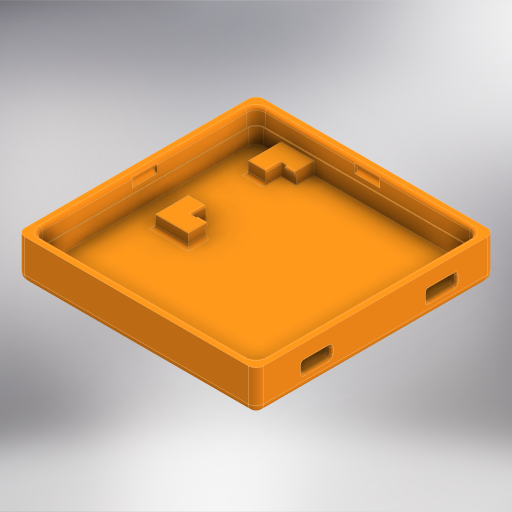
# Autodesk Inventor part: Bottom Plate
Saved by Autodesk Inventor 2024 (Build 280153000, 153)
## iProperties
Created: 2026-05-15
Part Number: Bottom Plate
Material: Generic
Document SubType Name: Modeling
Designer: Satyajit
Density: 1 g/cm^3
Appearance: Orange
Author: Satyajit
Autodesk Inventor part; units mm, degrees
ref_plane "YZ Plane" through (0, 0, 0) normal (1, 0, 0) x (0, 1, 0)
ref_plane "XZ Plane" through (0, 0, 0) normal (0, 1, 0) x (-1, 0, 0)
ref_plane "XY Plane" through (0, 0, 0) normal (0, 0, 1) x (1, 0, 0)
sketch "Sketch1" plane through (0, 0, 0) normal (0, 1, 0) x (-1, 0, 0)
  line L0 (35, -35) -> (-35, -35)
  line L1 (-35, -35) -> (-35, 35)
  line L2 (-35, 35) -> (35, 35)
  line L3 (35, 35) -> (35, -35)
  line L4 (35, -35) -> (-35, 35) construction
  line L5 (-35, -35) -> (35, 35) construction
  line L6 (-38, 38) -> (-38, -38)
  line L7 (-38, -38) -> (38, -38)
  line L8 (38, -38) -> (38, 38)
  line L9 (38, 38) -> (-38, 38)
  point P0 (0, 0)
  dimension "d0" = 70
  dimension "d1" = 3
  constraints: 20 end point, 4 parallel, 3 perpendicular, 2 midpoint, 1 horizontal, 3 other
  measures "d0" distance of L1.end L2.end
  measures "d1" distance between parallel lines of L1 L6
extrude "Extrusion1" add sketch "Sketch1" against normal blind 3 contours L0 L1 L2 L3 | L9 L8 L7 L6
extrude "Extrusion2" add sketch "Sketch1" along normal blind 10
sketch "Sketch2" plane through (0, 0, 0) normal (0, 1, 0) x (1, 0, 0)
  line L0 (-21, 29) -> (36, 29)
  line L1 (36, 29) -> (36, 1)
  line L2 (36, 1) -> (-21, 1)
  line L3 (-21, 1) -> (-21, 29) construction
  line L4 (-21, 29) -> (36, 1) construction
  line L5 (36, 29) -> (-21, 1) construction
  line L6 (-21, 24.15) -> (-27, 24.15) construction
  line L7 (-27, 24.15) -> (-27, 5.85) construction
  line L8 (-27, 5.85) -> (-21, 5.85) construction
  line L9 (35, 35) -> (35, -35) projected
  line L10 (-35, -35) -> (-35, 35) construction
  line L11 (38, 38) -> (38, -38) projected
  line L12 (-35, 35) -> (35, 35) projected
  line L13 (-21.4, 24.55) -> (-21.4, 29.4)
  line L14 (-21.4, 29.4) -> (-16.55, 29.4)
  line L15 (-16.55, 29.4) -> (-16.55, 35)
  line L16 (-21.4, 24.55) -> (-27, 24.55)
  line L17 (-27, 24.55) -> (-27, 35)
  line L18 (7.5, 15) -> (-27, 15) construction
  line L19 (-21.4, 5.45) -> (-21.4, 0.6)
  line L20 (-21.4, 0.6) -> (-16.55, 0.6)
  line L21 (-16.55, 0.6) -> (-16.55, -5)
  line L22 (-21.4, 5.45) -> (-27, 5.45)
  line L23 (-27, 5.45) -> (-27, -5)
  line L24 (-27, -5) -> (-16.55, -5)
  line L25 (35, 0.5) -> (36, 0.5)
  line L26 (36, 0.5) -> (36, 1)
  line L27 (35, 29) -> (35, 29.5)
  line L28 (35, 29.5) -> (36, 29.5)
  line L29 (36, 29.5) -> (36, 29)
  point P0 (0, 0)
  point P1 (40, 34)
  point P2 (35, 1)
  dimension "d16" = 57
  dimension "d17" = 28
  dimension "d18" = 6
  dimension "d19" = 18.3
  dimension "d26" = 2
  dimension "d27" = 6
  dimension "d28" = 0.4
  dimension "d29" = 0.4
  dimension "d30" = 0.4
  dimension "d35" = 0.5
  constraints: 52 end point, 11 perpendicular, 8 point on line, 6 symmetric about line, 4 horizontal, 3 midpoint, 2 collinear, 2 parallel, 1 horizontal alignment, 1 vertical, 1 other
  measures "d16" distance of L0.start L0.end
  measures "d17" distance of L0.end L1.end
  measures "d18" distance between parallel lines of L3 L7
  measures "d19" distance of L6.end L7.end
  measures "d26" distance between parallel lines of L11 L1
  measures "d27" distance between parallel lines of L12 L0
  measures "d28" distance between parallel lines of L6 L16
  measures "d29" distance between parallel lines of L13 L3
  measures "d30" distance between parallel lines of L14 L0
  measures "d35" distance of L28.end L0.end
extrude "Extrusion3" add sketch "Sketch2" along normal blind 4 contours L12 L15 L14 L13 L16 L17 | L19 L20 L21 L24 L23 L22
extrude "Extrusion4" cut sketch "Sketch2" along normal blind 6 contours L9 L28 L29 L0 | L0 L1 L2 L9 | L2 L26 L25 L9
sketch "Sketch3" plane through (36, 0, -29.5) normal (-1, 0, 0) x (0, 0, 1)
  line L0 (29, 0) -> (0, 0) projected
  line L1 (29, 0) -> (29, 6) projected
  line L2 (29, 6) -> (0, 6) projected
  line L3 (0, 0) -> (0, 6) projected
  line L4 (4.35, 1.45) -> (12.65, 1.45)
  line L5 (13.15, 1.95) -> (13.15, 4.45)
  line L6 (12.65, 4.95) -> (4.35, 4.95)
  line L7 (3.85, 4.45) -> (3.85, 1.95)
  line L8 (3.85, 1.45) -> (13.15, 4.95) construction
  line L9 (13.15, 1.45) -> (3.85, 4.95) construction
  line L10 (14.5, 0) -> (14.5, 6) construction
  line L11 (24.65, 1.45) -> (16.35, 1.45)
  line L12 (15.85, 1.95) -> (15.85, 4.45)
  line L13 (16.35, 4.95) -> (24.65, 4.95)
  line L14 (25.15, 4.45) -> (25.15, 1.95)
  line L15 (25.15, 1.45) -> (15.85, 4.95) construction
  line L16 (15.85, 1.45) -> (25.15, 4.95) construction
  arc A0 (3.85, 1.95) -> (4.35, 1.45) centre (4.35, 1.95) ccw
  arc A1 (4.35, 4.95) -> (3.85, 4.45) centre (4.35, 4.45) ccw
  arc A2 (13.15, 4.45) -> (12.65, 4.95) centre (12.65, 4.45) ccw
  arc A3 (12.65, 1.45) -> (13.15, 1.95) centre (12.65, 1.95) ccw
  arc A4 (15.85, 1.95) -> (16.35, 1.45) centre (16.35, 1.95) ccw
  arc A5 (16.35, 4.95) -> (15.85, 4.45) centre (16.35, 4.45) ccw
  arc A6 (25.15, 4.45) -> (24.65, 4.95) centre (24.65, 4.45) ccw
  arc A7 (24.65, 1.45) -> (25.15, 1.95) centre (24.65, 1.95) ccw
  line L17 (44.4, 1.45) -> (52.1, 1.45)
  line L18 (52.9, 2.25) -> (52.9, 4.15)
  line L19 (52.1, 4.95) -> (44.4, 4.95)
  line L20 (43.6, 4.15) -> (43.6, 2.25)
  line L21 (43.6, 1.45) -> (52.9, 4.95) construction
  line L22 (52.9, 1.45) -> (43.6, 4.95) construction
  arc A8 (43.6, 2.25) -> (44.4, 1.45) centre (44.4, 2.25) ccw
  arc A9 (44.4, 4.95) -> (43.6, 4.15) centre (44.4, 4.15) ccw
  arc A10 (52.9, 4.15) -> (52.1, 4.95) centre (52.1, 4.15) ccw
  arc A11 (52.1, 1.45) -> (52.9, 2.25) centre (52.1, 2.25) ccw
  line L23 (29, 0) -> (67.5, 0)
  line L24 (67.5, -3) -> (67.5, 10) projected
  line L25 (42.25, 0) -> (42.25, 6)
  line L26 (42.25, 6) -> (54.25, 6)
  line L27 (54.25, 6) -> (54.25, 0)
  point P0 (29.5, 0)
  point P1 (8.5, 3.2)
  point P2 (20.5, 3.2)
  point P3 (20.5, 3.2)
  point P4 (48.25, 3.2)
  point P5 (48.25, 0)
  point P6 (48.25, 6)
  dimension "d36" = 9.3
  dimension "d37" = 3.5
  dimension "d40" = 12
  dimension "d41" = 3.2
  dimension "d42" = 0.5
  dimension "d45" = 9.3
  dimension "d46" = 3.5
  dimension "d47" = 0.8
  dimension "d48" = 12
  constraints: 46 end point, 27 point on line, 24 point on circle, 24 tangent, 12 centre point, 10 equal radius, 9 midpoint, 5 parallel, 5 symmetric about line, 4 perpendicular, 3 horizontal, 2 vertical alignment, 1 horizontal alignment, 1 vertical
  measures "d36" distance of L8.end L9.end
  measures "d37" distance of L9.start L8.end
  measures "d40" distance of point (8.5, 3.2) point (20.5, 3.2)
  measures "d41" distance from line of L0 point (8.5, 3.2)
  measures "d42" radius of A0
  measures "d45" distance of L21.end L22.end
  measures "d46" distance of L22.start L21.end
  measures "d47" radius of A8
  measures "d48" distance between parallel lines of L27 L25
extrude "Extrusion5" cut sketch "Sketch3" against normal blind 6 contours A0 L7 A1 L6 A2 L5 A3 L4 | A8 L20 A9 L19 A10 L18 A11 L17
extrude "Extrusion6" cut sketch "Sketch3" along normal blind 6 contours A8 L20 A9 L19 A10 L18 A11 L17 | L25 L26 L27 L23
sketch "Sketch4" plane through (0, 4, 0) normal (0, 1, 0) x (1, 0, 0)
  line L0 (-16.55, 0.6) -> (-21.4, 0.6) projected
  line L1 (-21.4, 0.6) -> (-21.4, 5.45) projected
  line L2 (-16.55, -5) -> (-16.55, 0.6) projected
  line L3 (-16.55, 0.6) -> (-16.55, 1.3)
  line L4 (-16.55, 1.3) -> (-19.55, 1.3)
  line L5 (-19.55, 1.3) -> (-19.55, 0.6)
  line L6 (-21.4, 5.45) -> (-27, 5.45) projected
  line L7 (-27, 35) -> (-27, 24.55) projected
  line L8 (-27, 5.45) -> (-27, 24.55) construction
  line L9 (-27, 15) -> (0, 15) construction
  line L10 (-27, 24.55) -> (-21.4, 24.55) projected
  line L11 (-21.4, 24.55) -> (-21.4, 29.4) projected
  line L12 (-21.4, 29.4) -> (-16.55, 29.4) projected
  line L13 (-16.55, 29.4) -> (-16.55, 28.7)
  line L14 (-16.55, 28.7) -> (-19.55, 28.7)
  line L15 (-19.55, 28.7) -> (-19.55, 29.4)
  point P0 (0, 0)
  point P1 (-19.55, 29.4)
  dimension "d51" = 0.7
  dimension "d52" = 3
  constraints: 16 end point, 3 symmetric about line, 2 perpendicular, 2 vertical, 1 horizontal, 1 midpoint, 1 point on line, 1 vertical alignment
  measures "d51" distance of L0.start L3.end
  measures "d52" distance of L3.end L4.end
extrude "Extrusion7" add sketch "Sketch4" against normal blind 1
fillet "Fillet1" radius 0.5 4 edges at (-18.05, 4, -1.3) (-18.05, 3, -1.3) (-18.05, 4, -28.7) (-18.05, 3, -28.7)
fillet "Fillet2" radius 1 2 edges at (-18.05, 3, -0.6) (-18.05, 3, -29.4)
fillet "Fillet3" radius 0.5 8 edges at (-21.4, 4, -26.975) (-21.4, 4, -3.025) (35, 3, -29.5) (35, 6, -15) (35, 3, -0.5) (35, 3, 12.75) (35, 6, 18.75) (35, 3, 24.75)
fillet "Fillet4" radius 2.5 8 edges at (35, 5, -35) (38, 3.5, -38) (38, 3.5, 38) (35, 5, 35) (-38, 3.5, -38) (-38, 3.5, 38) (-35, 5, 35) (-35, 5, -35)
fillet "Fillet6" radius 1 5 edges at (-21.775, 0, 5) (-27, 0, -0.225) (-24.2, 0, -24.55) (-27, 0, -29.775) (-16.55, 0, 2.2)
fillet "Fillet7" radius 2.5 8 edges at (37.2678, -3, 37.2678) (0, -3, 38) (-37.2678, -3, 37.2678) (-38, -3, 0) (-37.2678, -3, -37.2678) (0, -3, -38) (37.2678, -3, -37.2678) (38, -3, 0)
sketch "Sketch5" plane through (0, 10, 0) normal (0, 1, 0) x (1, 0, 0)
  line L0 (-32.5, 35) -> (32.5, 35) projected
  arc A0 (-32.5, 35) -> (-35, 32.5) centre (-32.5, 32.5) ccw projected
  line L1 (-35, -32.5) -> (-35, 32.5) projected
  arc A1 (35, 32.5) -> (32.5, 35) centre (32.5, 32.5) ccw projected
  line L2 (35, 32.5) -> (35, -32.5) projected
  arc A2 (32.5, -35) -> (35, -32.5) centre (32.5, -32.5) ccw projected
  line L3 (32.5, -35) -> (-32.5, -35) projected
  arc A3 (-35, -32.5) -> (-32.5, -35) centre (-32.5, -32.5) ccw projected
  line L4 (32.5, 35.4) -> (-32.5, 35.4)
  arc A4 (-32.5, 35.4) -> (-35.4, 32.5) centre (-32.5, 32.5) ccw
  line L5 (-35.4, 32.5) -> (-35.4, -32.5)
  arc A5 (-35.4, -32.5) -> (-32.5, -35.4) centre (-32.5, -32.5) ccw
  line L6 (-32.5, -35.4) -> (32.5, -35.4)
  arc A6 (32.5, -35.4) -> (35.4, -32.5) centre (32.5, -32.5) ccw
  line L7 (35.4, -32.5) -> (35.4, 32.5)
  arc A7 (35.4, 32.5) -> (32.5, 35.4) centre (32.5, 32.5) ccw
  point P0 (0, 0)
  dimension "d62" = 0.4
  constraints: 8 end point, 8 point on circle, 4 centre point, 7 other
  measures "d62" distance between parallel lines of L0 L4
extrude "Extrusion8" cut sketch "Sketch5" against normal blind 5
fillet "Fillet8" radius 0.6 16 edges at (38, 1.6843, 23.1657) (38, 3.2, 23.4) (38, 4.7157, 23.1657) (38, 4.95, 18.75) (38, 4.7157, 14.3343) (38, 3.2, 14.1) (38, 1.6843, 14.3343) (38, 1.45, 18.75) (38, 1.5964, -16.4964) (38, 3.2, -16.35) (38, 4.8036, -16.4964) (38, 4.95, -21) (38, 4.8036, -25.5036) (38, 3.2, -25.65) (38, 1.5964, -25.5036) (38, 1.45, -21)
sketch "Sketch6" plane through (0, 0, 0) normal (0, 0, 1) x (1, 0, 0)
  line L0 (-35.4, 10) -> (-35.4, 5) projected
  circle A0 centre (-35.4, 7.5) radius 1
  point P0 (0, 0)
  point P1 (-35.4, 6.5)
  dimension "d66" = 2
  dimension "d73" = 2.5
  constraints: 1 centre point, 1 midpoint
  measures "d66" diameter of A0
  measures "d73" distance of L0.start A0.centre
extrude "Extrusion9" cut sketch "Sketch6" along normal mid plane 8
pattern_circular "Circular Pattern1" count 4 over 360 about axis through (0, -10, 0) along (0, 1, 0) of "Extrusion9"
fillet "Fillet10" radius 1 8 edges at (34.5506, 10, -34.5506) (35.4, 10, 0) (34.5506, 10, 34.5506) (0, 10, 35.4) (-34.5506, 10, 34.5506) (-35.4, 10, 0) (-34.5506, 10, -34.5506) (0, 10, -35.4)
fillet "Fillet11" radius 0.8 4 edges at (-35.4, 8.5, 0) (0, 8.5, -35.4) (35.4, 8.5, 0) (0, 8.5, 35.4)
body "Solid1"
